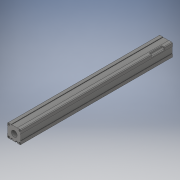
# Autodesk Inventor part: 1470874 EPCO-25-30000_z---(0)
Saved by Autodesk Inventor 2019 (Build 230136000, 136)
## iProperties
Created: 2023-04-07
Part Number: 1470874 EPCO-25-30000_z---(0)
Material: Generic
Catalog Web Link: www.cadenas.de
Description: EPCO_z-electric cylinder
Vendor: FESTO
Document SubType Name: Modeling
Designer: psAdmin
Manufacturer: FESTO
Mass: 404.951 g
Surface Area: 1289.21 cm^2
Volume: 404.951 cm^3
Density: 1 g/cm^3
Appearance: PSOLRGB-128-128-128
Category: PARTsolutions
Company: FESTO
Title: 1470874 EPCO-25-30000_z---(0)
Author: Cadenas PARTsolutions
Comments: electric cylinder
PSOL_IDENT_0: {$CADENAS_DATA/23d-libs/festo/parts/e/epco/parts/epco_z.prj},220 {VTYP=3D},{NB=1470874 EPCO-25-30000
PSOL_IDENT_1: _z---(0)},{LINA=1470874 EPCO-25-30000_z---(0)},{NN=EPCO_z},{DATE=16.03.2023 11:34:06},{GEOMDATE=16.0
PSOL_IDENT_2: 3.2023 11:30:21},{VERSION=},{LINEID=20},{WBVAR=HUB,OA,KOLB},{WBNUMERIC=HUB,OA,KOLB}  {NB=1470874 EPC
PSOL_IDENT_3: O-25-30000_z---(0)},{LINA=1470874 EPCO-25-30000_z---(0)},{KT=DUMMY},{TNR=1470874},{TYP=EPCO-25},{KDM=
PSOL_IDENT_4: 25},{HUB=300},{OA=0},{KOLB=0},{B1=40.000},{B2=32.500},{RA=31.000},{B5=18.000},{L2=156.600},{B6=14.00
PSOL_IDENT_5: 0},{D3N=5.000},{LK=62.600},{LX1=22.000},{LX2=20.000},{RX=8.000},{LK1=38.100},{BM2=31.000},{DK1=6.000
PSOL_IDENT_6: },{DK2=3.400},{LK2=41.600},{D4=22.000},{L7=2.500},{L8=4.600},{D5=5.000},{D1=17.270},{L6=12.000},{L4=
PSOL_IDENT_7: 18.000},{ROT=0}
NB: 1470874 EPCO-25-30000_z---(0)
NN: EPCO_z
NT: electric cylinder
NBSYN: $TNR. $TYP.-$HUB.$OA.$KOLB._z---($ROT.)
LINA: 1470874 EPCO-25-30000_z---(0)
CATALOG: Festo
TNR: 1470874
TYP: EPCO-25
KDM: 25
HUB: 300
OA: -
KOLB: 0
B1: 40
B2: 32.5
RA: 31
B5: 18
L2: 156.6
B6: 14
D3N: 5
LK: 62.6
LX1: 22
LX2: 20
RX: 8
LK1: 38.1
BM2: 31
DK1: 6
DK2: 3.4
LK2: 41.6
D4: 22
L7: 2.5
L8: 4.6
D5: 5
D1: 17.27
L6: 12
L4: 18
SUPPLIER: FESTO
ARTICLENO: 1470874 EPCO-25-30000_z---(0)
BOMINFO: 1470874 EPCO-25-30000_z---(0)
CREATOR: CADENAS GmbH
Autodesk Inventor part; units mm, degrees
sketch "Sketch_1" plane through (0, 0, 0) normal (0, 0, 1) x (1, 0, 0)
  arc A0 (-20, -18) -> (-18, -20) centre (-18, -18) ccw
  line L0 (-18, -20) -> (18, -20)
  arc A1 (18, -20) -> (20, -18) centre (18, -18) ccw
  line L1 (20, -18) -> (20, 18)
  arc A2 (20, 18) -> (18, 20) centre (18, 18) ccw
  line L2 (18, 20) -> (-18, 20)
  arc A3 (-18, 20) -> (-20, 18) centre (-18, 18) ccw
  line L3 (-20, 18) -> (-20, -18)
  constraints: 8 end point, 8 point on circle, 4 centre point
extrude "Extrusion1" add sketch "Sketch_1" against normal blind 456.6
sketch "Sketch_2" plane through (0, 0, 0) normal (0, 0, 1) x (1, 0, 0)
  line L0 (-40, -40) -> (40, -40)
  line L1 (40, -40) -> (40, 40)
  line L2 (40, 40) -> (-40, 40)
  line L3 (-40, 40) -> (-40, -40)
  arc A0 (-18.8146, 8.4904) -> (-18.8146, -8.4904) centre (11, 0) ccw
  arc A1 (-19.1993, -9) -> (-18.8146, -8.4904) centre (-19.1993, -8.6) ccw
  line L4 (-19.1993, -9) -> (-19.8, -9)
  arc A2 (-19.8, -9) -> (-20, -9.2) centre (-19.8, -9.2) ccw
  line L5 (-20, -9.2) -> (-20, -18)
  arc A3 (-20, -18) -> (-18, -20) centre (-18, -18) ccw
  line L6 (-18, -20) -> (-9.25, -20)
  line L7 (-9.25, -20) -> (-8.5879, -19.3379)
  arc A4 (-8.5879, -19.3379) -> (-8.5, -19.1257) centre (-8.8, -19.1257) ccw
  line L8 (-8.5, -19.1257) -> (-8.5, -19)
  arc A5 (-8.5, -19) -> (-8.8, -18.7) centre (-8.8, -19) ccw
  line L9 (-8.8, -18.7) -> (-9.9986, -18.7)
  arc A6 (-10.3168, -17.9318) -> (-9.9986, -18.7) centre (-9.9986, -18.25) ccw
  line L10 (-10.3168, -17.9318) -> (-8.8122, -16.4272)
  arc A7 (-7.5394, -15.9) -> (-8.8122, -16.4272) centre (-7.5394, -17.7) ccw
  line L11 (-7.5394, -15.9) -> (-6.4606, -15.9)
  arc A8 (-5.1878, -16.4272) -> (-6.4606, -15.9) centre (-6.4606, -17.7) ccw
  line L12 (-5.1878, -16.4272) -> (-3.6832, -17.9318)
  arc A9 (-4.0014, -18.7) -> (-3.6832, -17.9318) centre (-4.0014, -18.25) ccw
  line L13 (-4.0014, -18.7) -> (-5.2, -18.7)
  arc A10 (-5.2, -18.7) -> (-5.5, -19) centre (-5.2, -19) ccw
  line L14 (-5.5, -19) -> (-5.5, -19.1257)
  arc A11 (-5.5, -19.1257) -> (-5.4121, -19.3379) centre (-5.2, -19.1257) ccw
  line L15 (-5.4121, -19.3379) -> (-4.75, -20)
  line L16 (-4.75, -20) -> (4.75, -20)
  line L17 (4.75, -20) -> (5.4121, -19.3379)
  arc A12 (5.4121, -19.3379) -> (5.5, -19.1257) centre (5.2, -19.1257) ccw
  line L18 (5.5, -19.1257) -> (5.5, -19)
  arc A13 (5.5, -19) -> (5.2, -18.7) centre (5.2, -19) ccw
  line L19 (5.2, -18.7) -> (4.0014, -18.7)
  arc A14 (3.6832, -17.9318) -> (4.0014, -18.7) centre (4.0014, -18.25) ccw
  line L20 (3.6832, -17.9318) -> (5.1878, -16.4272)
  arc A15 (6.4606, -15.9) -> (5.1878, -16.4272) centre (6.4606, -17.7) ccw
  line L21 (6.4606, -15.9) -> (7.5394, -15.9)
  arc A16 (8.8122, -16.4272) -> (7.5394, -15.9) centre (7.5394, -17.7) ccw
  line L22 (8.8122, -16.4272) -> (10.3168, -17.9318)
  arc A17 (9.9986, -18.7) -> (10.3168, -17.9318) centre (9.9986, -18.25) ccw
  line L23 (9.9986, -18.7) -> (8.8, -18.7)
  arc A18 (8.8, -18.7) -> (8.5, -19) centre (8.8, -19) ccw
  line L24 (8.5, -19) -> (8.5, -19.1257)
  arc A19 (8.5, -19.1257) -> (8.5879, -19.3379) centre (8.8, -19.1257) ccw
  line L25 (8.5879, -19.3379) -> (9.25, -20)
  line L26 (9.25, -20) -> (18, -20)
  arc A20 (18, -20) -> (20, -18) centre (18, -18) ccw
  line L27 (20, -18) -> (20, -9.2)
  arc A21 (20, -9.2) -> (19.8, -9) centre (19.8, -9.2) ccw
  line L28 (19.8, -9) -> (19.1993, -9)
  arc A22 (18.8146, -8.4904) -> (19.1993, -9) centre (19.1993, -8.6) ccw
  arc A23 (18.8146, -8.4904) -> (18.8146, 8.4904) centre (-11, 0) ccw
  arc A24 (19.1993, 9) -> (18.8146, 8.4904) centre (19.1993, 8.6) ccw
  line L29 (19.1993, 9) -> (19.8, 9)
  arc A25 (19.8, 9) -> (20, 9.2) centre (19.8, 9.2) ccw
  line L30 (20, 9.2) -> (20, 18)
  arc A26 (20, 18) -> (18, 20) centre (18, 18) ccw
  line L31 (18, 20) -> (9.2, 20)
  arc A27 (9.2, 20) -> (9, 19.8) centre (9.2, 19.8) ccw
  line L32 (9, 19.8) -> (9, 19.1993)
  arc A28 (8.4904, 18.8146) -> (9, 19.1993) centre (8.6, 19.1993) ccw
  arc A29 (8.4904, 18.8146) -> (-8.4904, 18.8146) centre (0, -11) ccw
  arc A30 (-9, 19.1993) -> (-8.4904, 18.8146) centre (-8.6, 19.1993) ccw
  line L33 (-9, 19.1993) -> (-9, 19.8)
  arc A31 (-9, 19.8) -> (-9.2, 20) centre (-9.2, 19.8) ccw
  line L34 (-9.2, 20) -> (-18, 20)
  arc A32 (-18, 20) -> (-20, 18) centre (-18, 18) ccw
  line L35 (-20, 18) -> (-20, 9.2)
  arc A33 (-20, 9.2) -> (-19.8, 9) centre (-19.8, 9.2) ccw
  line L36 (-19.8, 9) -> (-19.1993, 9)
  arc A34 (-18.8146, 8.4904) -> (-19.1993, 9) centre (-19.1993, 8.6) ccw
  constraints: 74 end point, 70 point on circle, 35 centre point
extrude "Extrusion2" cut sketch "Sketch_2" against normal blind 456.6
sketch "Sketch_3" plane through (0, 0, -394) normal (0, 0, 1) x (1, 0, 0)
  line L0 (-40, -40) -> (40, -40)
  line L1 (40, -40) -> (40, 40)
  line L2 (40, 40) -> (-40, 40)
  line L3 (-40, 40) -> (-40, -40)
  arc A0 (-14.0156, -19.5) -> (-20, -12.254) centre (-22, -20) ccw
  line L4 (-14.0156, -19.5) -> (-13.5156, -20)
  line L5 (-13.5156, -20) -> (20, -20)
  line L6 (20, -20) -> (20, 12.254)
  arc A1 (15.4322, 15.4322) -> (20, 12.254) centre (22, 20) ccw
  arc A2 (12.254, 20) -> (15.4322, 15.4322) centre (20, 22) ccw
  line L7 (12.254, 20) -> (-20, 20)
  line L8 (-20, 20) -> (-20, -12.254)
  constraints: 18 end point, 6 point on circle, 3 centre point
extrude "Extrusion3" cut sketch "Sketch_3" against normal blind 38.1
sketch "Sketch_4" plane through (-15.5, 0, 0) normal (1, 0, 0) x (0, 0, -1)
  line L0 (456.6, -15.5) -> (394, -15.5)
  line L1 (394, -15.5) -> (394, -12.5)
  line L2 (394, -12.5) -> (435.6, -12.5)
  line L3 (435.6, -12.5) -> (435.6, -13.8)
  line L4 (435.6, -13.8) -> (456.6, -13.8)
  line L5 (456.6, -13.8) -> (456.6, -15.5)
  line L6 (456.6, -15.5) -> (394, -15.5)
  constraints: 14 end point
revolve "Revolution1" cut sketch "Sketch_4" angle 360 about axis through (-15.5, -15.5, -456.6) along (0, 0, -1)
sketch "Sketch_5" plane through (15.5, 0, 0) normal (1, 0, 0) x (0, 0, -1)
  line L0 (456.6, 15.5) -> (394, 15.5)
  line L1 (394, 15.5) -> (394, 18.5)
  line L2 (394, 18.5) -> (435.6, 18.5)
  line L3 (435.6, 18.5) -> (435.6, 17.2)
  line L4 (435.6, 17.2) -> (456.6, 17.2)
  line L5 (456.6, 17.2) -> (456.6, 15.5)
  line L6 (456.6, 15.5) -> (394, 15.5)
  constraints: 14 end point
revolve "Revolution2" cut sketch "Sketch_5" angle 360 about axis through (15.5, 15.5, -456.6) along (0, 0, -1)
sketch "Sketch_6" plane through (0, 0, 0) normal (1, 0, 0) x (0, 1, 0)
  line L0 (0, -456.6) -> (0, -442)
  line L1 (0, -442) -> (2.5, -442)
  line L2 (2.5, -442) -> (2.5, -452)
  line L3 (2.5, -452) -> (6.8, -452)
  line L4 (6.8, -452) -> (7, -451.8)
  line L5 (7, -451.8) -> (7, -442)
  line L6 (7, -442) -> (9.5, -442)
  line L7 (9.5, -442) -> (9.5, -454.1)
  line L8 (9.5, -454.1) -> (11, -454.1)
  line L9 (11, -454.1) -> (11, -456.6)
  line L10 (11, -456.6) -> (0, -456.6)
  line L11 (0, -456.6) -> (0, -442)
  constraints: 24 end point
revolve "Revolution3" cut sketch "Sketch_6" angle 360 about axis through (0, 0, -456.6) along (0, 0, -1)
sketch "Sketch_7" plane through (0, 0, 0) normal (1, 0, 0) x (0, 1, 0)
  line L0 (0, -384) -> (0, 18)
  line L1 (0, 18) -> (8.635, 18)
  line L2 (8.635, 18) -> (8.635, -74)
  line L3 (8.635, -74) -> (16.6667, -74)
  line L4 (16.6667, -74) -> (16.6667, -384)
  line L5 (16.6667, -384) -> (0, -384)
  line L6 (0, -384) -> (0, 18)
  constraints: 14 end point
revolve "Revolution4" cut sketch "Sketch_7" angle 360 about axis through (0, 0, -384) along (0, 0, -1)
sketch "Sketch8" plane through (0, 0, 0) normal (0, 0, 1) x (1, 0, 0)
  point P0 (16.25, 16.25)
hole "Hole1" at (16.25, 16.25, 0) direction (0, 0, -1) diameter 4.134 depth 14 tip angle 120 countersink diameter 5 countersink angle 90 thread size "M5x0.8" class "6H" standard "ISO Metric profile"
sketch "Sketch9" plane through (0, 0, 0) normal (0, 0, 1) x (1, 0, 0)
  point P0 (16.25, -16.25)
hole "Hole2" at (16.25, -16.25, 0) direction (0, 0, -1) diameter 4.134 depth 14 tip angle 120 countersink diameter 5 countersink angle 90 thread size "M5x0.8" class "6H" standard "ISO Metric profile"
sketch "Sketch10" plane through (0, 0, 0) normal (0, 0, 1) x (1, 0, 0)
  point P0 (-16.25, 16.25)
hole "Hole3" at (-16.25, 16.25, 0) direction (0, 0, -1) diameter 4.134 depth 14 tip angle 120 countersink diameter 5 countersink angle 90 thread size "M5x0.8" class "6H" standard "ISO Metric profile"
sketch "Sketch11" plane through (0, 0, 0) normal (0, 0, 1) x (1, 0, 0)
  point P0 (-16.25, -16.25)
hole "Hole4" at (-16.25, -16.25, 0) direction (0, 0, -1) diameter 4.134 depth 14 tip angle 120 countersink diameter 5 countersink angle 90 thread size "M5x0.8" class "6H" standard "ISO Metric profile"
ref_plane "ANBAU_XY" through (0, 0, 0) normal (0, 0, -1) x (1, 0, 0)
ref_plane "ANBAU_YZ" through (0, 0, 0) normal (1, 0, 0) x (0, -1, 0)
ref_plane "ANBAU_ZX" through (0, 0, 0) normal (0, -1, 0) x (0, 0, -1)
ref_plane "DIM_H2_2_XY" through (18, -20, 0) normal (0, 0, 1) x (1, 0, 0)
ref_plane "DIM_H2_2_YZ" through (18, -20, 0) normal (1, 0, 0) x (0, 1, 0)
ref_plane "DIM_H2_2_ZX" through (18, -20, 0) normal (0, 1, 0) x (0, 0, 1)
ref_plane "SCREW_1_XY" through (15.5, 15.5, -435.6) normal (0, 0, -1) x (1, 0, 0)
ref_plane "SCREW_1_YZ" through (15.5, 15.5, -435.6) normal (1, 0, 0) x (0, -1, 0)
ref_plane "SCREW_1_ZX" through (15.5, 15.5, -435.6) normal (0, -1, 0) x (0, 0, -1)
ref_plane "SCREW_2_XY" through (-15.5, -15.5, -435.6) normal (0, 0, -1) x (1, 0, 0)
ref_plane "SCREW_2_YZ" through (-15.5, -15.5, -435.6) normal (1, 0, 0) x (0, -1, 0)
ref_plane "SCREW_2_ZX" through (-15.5, -15.5, -435.6) normal (0, -1, 0) x (0, 0, -1)
ref_plane "TO_KS_XY" through (0, 0, 0) normal (0, 0, 1) x (1, 0, 0)
ref_plane "TO_KS_YZ" through (0, 0, 0) normal (1, 0, 0) x (0, 1, 0)
ref_plane "TO_KS_ZX" through (0, 0, 0) normal (0, 1, 0) x (0, 0, 1)
ref_plane "TO_MOTOR_XY" through (0, 0, -456.6) normal (0, 0, 1) x (1, 0, 0)
ref_plane "TO_MOTOR_YZ" through (0, 0, -456.6) normal (1, 0, 0) x (0, 1, 0)
ref_plane "TO_MOTOR_ZX" through (0, 0, -456.6) normal (0, 1, 0) x (0, 0, 1)
body "Solid1"
